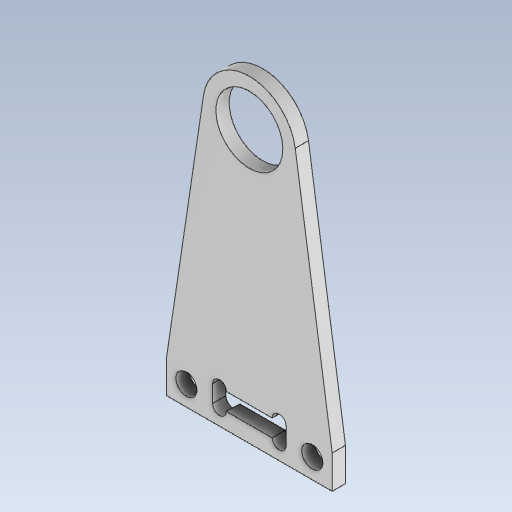
# Autodesk Inventor part: Foot_front_frame
Saved by Autodesk Inventor 2020.4 (Build 244396000, 396)
## iProperties
Part Number: Foot_front_frame
Material: アルミニウム 2014-T4
Document SubType Name: Modeling
Designer: Masato Kubotera
Density: 2.8 g/cm^3
Appearance: 滑らか - 淡い灰色
Description: A2017 T2
Mass: 4.3393 g
Surface Area: 19.7745 cm^2
Volume: 1.54975 cm^3
Author: Masato Kubotera
Autodesk Inventor part; units mm, degrees
ref_plane "YZ Plane" through (0, 0, 0) normal (1, 0, 0) x (0, 1, 0)
ref_plane "XZ Plane" through (0, 0, 0) normal (0, 1, 0) x (-1, 0, 0)
ref_plane "XY Plane" through (0, 0, 0) normal (0, 0, 1) x (1, 0, 0)
derived "Foot_back_frame.ipt"
sketch "スケッチ1" plane through (0, 0, 0) normal (1, 0, 0) x (0, 1, 0)
  circle A0 centre (0, 0) radius 5.05
  line L0 (-10.9106, 0) -> (10.9106, 0) construction
  line L1 (0, 11.25) -> (0, -41) construction
  line L2 (-10.8894, 0.4808) -> (-12.5, -36)
  line L3 (-12.5, -36) -> (-12.5, -41)
  line L4 (-12.5, -41) -> (12.5, -41)
  circle A1 centre (0, 8.5) radius 1.35
  circle A2 centre (0, 8.5) radius 2.4 construction
  circle A3 centre (-8.5, 0) radius 1.35
  circle A4 centre (0, -8.5) radius 1.35
  circle A5 centre (8.5, 0) radius 1.35
  line L5 (5.5, -36) -> (-5.5, -36) construction
  line L6 (-5.5, -36) -> (-5.5, -38.5) construction
  line L7 (-5.5, -38.5) -> (5.5, -38.5) construction
  line L8 (5.5, -38.5) -> (5.5, -36) construction
  line L9 (5.5, -36) -> (-5.5, -38.5) construction
  line L10 (-5.5, -36) -> (5.5, -38.5) construction
  circle A6 centre (-9.5, -38) radius 1.6
  line L11 (-12.5, -38) -> (12.1081, -38) construction
  circle A7 centre (-9.5, -38) radius 2.75 construction
  line L12 (-5.55, -35.95) -> (5.55, -35.95)
  line L13 (5.55, -35.95) -> (5.55, -38.55)
  line L14 (5.55, -38.55) -> (-5.55, -38.55)
  line L15 (-5.55, -38.55) -> (-5.55, -35.95)
  line L16 (-5.55, -35.95) -> (5.55, -38.55) construction
  line L17 (5.55, -35.95) -> (-5.55, -38.55) construction
  arc A8 (-3.45, -35.95) -> (-5.55, -35.95) centre (-4.5, -35.95) ccw
  line L18 (-5.5, -37.25) -> (5.5, -37.25) construction
  arc A9 (-5.55, -38.55) -> (-3.45, -38.55) centre (-4.5, -38.55) ccw
  circle A10 centre (9.5, -38) radius 2.75 construction
  circle A11 centre (9.5, -38) radius 1.6
  arc A12 (5.55, -35.95) -> (3.45, -35.95) centre (4.5, -35.95) ccw
  arc A13 (3.45, -38.55) -> (5.55, -38.55) centre (4.5, -38.55) ccw
  line L19 (10.8894, 0.4808) -> (12.5, -36)
  line L20 (12.5, -36) -> (12.5, -41)
  arc A14 (10.8894, 0.4808) -> (-10.8894, 0.4808) centre (0, 0) ccw
  line L21 (-13.5, 1) -> (13.5, 1) construction
  circle A15 centre (-13.5, 1) radius 2.4 construction
  point P0 (0, -37.25)
  point P1 (0, 1)
sketch "スケッチ2" plane through (0, 0, 0) normal (1, 0, 0) x (0, 1, 0)
  circle A0 centre (0, 0) radius 5.05 projected
  circle A1 centre (0, 0) radius 4.05
  line L0 (-5.55, -35.95) -> (5.55, -35.95) projected
  arc A2 (-3.45, -35.95) -> (-5.55, -35.95) centre (-4.5, -35.95) ccw projected
  line L1 (-5.55, -38.55) -> (-5.55, -35.95) projected
  arc A3 (-5.55, -38.55) -> (-3.45, -38.55) centre (-4.5, -38.55) ccw projected
  line L2 (5.55, -38.55) -> (-5.55, -38.55) projected
  arc A4 (5.55, -35.95) -> (3.45, -35.95) centre (4.5, -35.95) ccw projected
  line L3 (5.55, -35.95) -> (5.55, -38.55) projected
  arc A5 (3.45, -38.55) -> (5.55, -38.55) centre (4.5, -38.55) ccw projected
  circle A6 centre (-9.5, -38) radius 1.6 projected
  circle A7 centre (9.5, -38) radius 1.6 projected
  line L4 (-12.5, -36) -> (-12.5, -41) projected
  line L5 (-12.5, -41) -> (12.5, -41) projected
  line L6 (12.5, -36) -> (12.5, -41) projected
  line L7 (-12.5, -36) -> (-6.922, 1.0423)
  arc A8 (6.922, 1.0423) -> (-6.922, 1.0423) centre (0, 0) ccw
  line L8 (0, 11.25) -> (0, -41) construction
  line L9 (12.5, -36) -> (6.922, 1.0423)
  dimension "d1" = 8.1
  dimension "d2" = 7
  constraints: 4 end point, 2 centre point, 2 concentric, 2 point on circle, 1 symmetric about line, 1 tangent
  measures "d1" diameter of A1
  measures "d2" radius of A8
extrude "押し出し1" add sketch "スケッチ2" along normal blind 2 contours L7 A8 L9 L6 L5 L4
